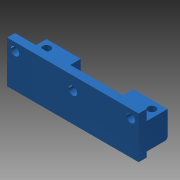
# Autodesk Inventor part: z endcap
Saved by Autodesk Inventor 2013 SP2 (Build 170200200, 200)
## iProperties
Created: 2017-05-18
Part Number: z endcap
Material: Generic
Document SubType Name: Modeling
Designer: Herman de Vries
Density: 1 g/cm^3
Author: Herman de Vries
Autodesk Inventor part; units mm, degrees
ref_plane "YZ Plane" through (0, 0, 0) normal (1, 0, 0) x (0, 1, 0)
ref_plane "XZ Plane" through (0, 0, 0) normal (0, 1, 0) x (-1, 0, 0)
ref_plane "XY Plane" through (0, 0, 0) normal (0, 0, 1) x (1, 0, 0)
sketch "Sketch1" plane through (0, 0, 0) normal (0, 0, 1) x (1, 0, 0)
  line L0 (0, 0) -> (46, 0)
  line L1 (46, 0) -> (46, 10)
  line L2 (46, 10) -> (0, 10)
  line L3 (0, 10) -> (0, 0)
  circle A0 centre (3, 7) radius 1.5
  circle A1 centre (43, 7) radius 1.5
  circle A2 centre (13, 3) radius 3
  circle A3 centre (33, 3) radius 3
  line L4 (18, 7) -> (28, 7)
  line L5 (28, 7) -> (28, 4)
  line L6 (28, 4) -> (18, 4)
  line L7 (18, 4) -> (18, 7)
  point P0 (23, 7)
  point P1 (23, 10)
  dimension "d2" = 10
  dimension "d3" = 3
  dimension "d4" = 3
  dimension "d5" = 3
  dimension "d6" = 3
  dimension "d7" = 3
  dimension "d8" = 40
  dimension "d11" = 6
  dimension "d12" = 6
  dimension "d13" = 10
  dimension "d14" = 10
  dimension "d26" = 7
  dimension "d27" = 10
  dimension "d28" = 3
  constraints: 16 end point, 4 centre point, 4 parallel, 3 horizontal alignment, 2 horizontal, 2 midpoint, 2 perpendicular, 1 vertical alignment
  measures "d2" distance of L2.end L0.start
  measures "d3" diameter of A0
  measures "d4" diameter of A1
  measures "d5" horizontal distance of A0.centre L2.end
  measures "d6" distance from line of L3 A0.centre
  measures "d7" distance from line of L1 A1.centre
  measures "d8" distance of A1.centre A0.centre
  measures "d11" diameter of A2
  measures "d12" diameter of A3
  measures "d13" horizontal distance of A0.centre A2.centre
  measures "d14" horizontal distance of A1.centre A3.centre
  measures "d26" distance from line of L2 A2.centre
  measures "d27" distance of L5.end L6.end
  measures "d28" distance of L4.end L5.end
extrude "Extrusion1" add sketch "Sketch1" along normal blind 10 contours A2 | A3 | L3 L2 L1 L0
sketch "Sketch2" plane through (0, 0, 10) normal (0, 0, 1) x (1, 0, 0)
  line L0 (46, 10) -> (0, 10) projected
  line L1 (0, 0) -> (46, 0) projected
  line L2 (13, 10) -> (33, 10)
  line L3 (33, 10) -> (33, 0)
  line L4 (33, 0) -> (13, 0)
  line L5 (13, 0) -> (13, 10)
  point P0 (23, 10)
  point P1 (23, 10)
  dimension "d15" = 20
  constraints: 8 end point, 2 midpoint, 2 parallel, 2 point on line, 1 coincident, 1 horizontal, 1 perpendicular
  measures "d15" distance of L2.start L2.end
extrude "Extrusion2" cut sketch "Sketch2" against normal blind 5
sketch "Sketch3" plane through (0, 0, 0) normal (0, -1, 0) x (1, 0, 0)
  line L0 (-2, 16) -> (48, 16)
  line L1 (48, 16) -> (48, 0)
  line L2 (48, 0) -> (-2, 0)
  line L3 (-2, 0) -> (-2, 16)
  line L4 (0, 10) -> (13, 10) projected
  line L5 (0, 0) -> (0, 10) projected
  line L6 (46, 0) -> (46, 10) projected
  line L7 (0, 0) -> (46, 0) projected
  point P0 (23, 16)
  point P1 (23, 0)
  dimension "d19" = 6
  dimension "d22" = 0
  dimension "d30" = 50
  constraints: 8 end point, 2 midpoint, 2 parallel, 1 horizontal, 1 perpendicular, 1 vertical alignment
  measures "d19" distance between parallel lines of L4 L0
  measures "d22" distance from line of L2 L6.start
  measures "d30" distance of L0.start L0.end
extrude "Extrusion3" add sketch "Sketch3" along normal blind 3
fillet "Fillet1" radius 1 4 edges at (23, 10, 5) (23, 10, 0) (23, 7, 0) (23, 7, 5)
sketch "Sketch4" plane through (0, -3, 0) normal (0, -1, 0) x (1, 0, 0)
  circle A0 centre (1, 13) radius 1.6
  circle A1 centre (45, 13) radius 1.6
  line L0 (48, 16) -> (-2, 16) projected
  circle A2 centre (23, 11) radius 1.6
  point P0 (0, 0)
  point P1 (23, 16)
  dimension "d32" = 3.2
  dimension "d33" = 3.2
  dimension "d34" = 3
  dimension "d35" = 3
  dimension "d36" = 3
  dimension "d37" = 3
  dimension "d38" = 3.2
  dimension "d39" = 5
  constraints: 3 centre point, 1 midpoint, 1 vertical alignment
  measures "d32" diameter of A0
  measures "d33" diameter of A1
  measures "d34" distance from line of L0 A0.centre
  measures "d35" horizontal distance of A1.centre L0.start
  measures "d36" horizontal distance of L0.start A1.centre
  measures "d37" horizontal distance of A0.centre L0.end
  measures "d38" diameter of A2
  measures "d39" vertical distance of A2.centre L0.end
extrude "Extrusion4" cut sketch "Sketch4" against normal blind 10
equation "\"d11\" = d12"
equation "\"d19\" = d20"
equation "\"d32\" = d38"
equation "\"d33\" = d38"
equation "\"d20\" = 6"
body "Solid1"
